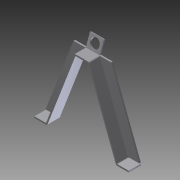
# Autodesk Inventor part: bunny throw base 2
Saved by Autodesk Inventor 2012 (Build 160160000, 160)
## iProperties
Created: 2013-10-11
Part Number: bunny throw base 2
Material: Default
Document SubType Name: Modeling
Designer: Bryce
Density: 1 g/cm^3
Author: Bryce
Autodesk Inventor part; units mm, degrees
ref_plane "YZ Plane" through (0, 0, 0) normal (1, 0, 0) x (0, 1, 0)
ref_plane "XZ Plane" through (0, 0, 0) normal (0, 1, 0) x (-1, 0, 0)
ref_plane "XY Plane" through (0, 0, 0) normal (0, 0, 1) x (1, 0, 0)
sketch "Sketch1" plane through (0, 0, 0) normal (0, 0, 1) x (1, 0, 0)
  line L0 (0, 0) -> (193.675, 0)
  line L1 (84.1375, 152.4) -> (109.5375, 152.4)
  line L2 (84.1375, 152.4) -> (25.9752, 0)
  line L3 (109.5375, 152.4) -> (167.6998, 0)
  line L4 (58.1623, 155.575) -> (0.6059, 4.7625)
  line L5 (135.5127, 155.575) -> (193.0691, 4.7625)
  line L6 (0, 0) -> (0, 3.175)
  line L7 (0, 3.175) -> (23.7885, 3.175)
  line L8 (193.675, 0) -> (193.675, 3.175)
  line L9 (193.675, 3.175) -> (169.8865, 3.175)
  line L10 (169.8865, 3.175) -> (111.7241, 155.575)
  line L11 (111.7241, 155.575) -> (81.9509, 155.575)
  line L12 (81.9509, 155.575) -> (23.7885, 3.175)
  line L13 (58.1623, 155.575) -> (81.9509, 155.575)
  line L14 (111.7241, 155.575) -> (135.5127, 155.575)
  line L15 (0.6059, 4.7625) -> (22.3923, 4.7625)
  line L16 (193.0691, 4.7625) -> (171.2827, 4.7625)
  arc A0 (22.3923, 3.175) -> (22.3923, 4.7625) centre (22.3923, 3.9688) ccw
  arc A1 (171.2827, 4.7625) -> (171.2827, 3.175) centre (171.2827, 3.9688) ccw
  dimension "d0" = 193.675
  dimension "d1" = 25.4
  dimension "d2" = 25.4
  dimension "d3" = 25.4
  dimension "d4" = 3.175
  dimension "d5" = 3.175
  dimension "d6" = 152.4
  dimension "d7" = 1.5875
  dimension "d8" = 1.5875
  dimension "d9" = 1.5875
  constraints: 34 end point, 8 point on line, 4 parallel, 4 perpendicular, 4 point on circle, 4 tangent, 3 collinear, 2 centre point, 2 horizontal alignment, 1 equal length, 1 horizontal, 2 other
  measures "d0" distance of L0.start L0.end
  measures "d1" distance of L1.start L1.end
  measures "d2" distance between parallel lines of L2 L4
  measures "d3" distance between parallel lines of L5 L3
  measures "d4" distance of L0.start L6.end
  measures "d5" distance between parallel lines of L11 L1
  measures "d6" distance between parallel lines of L0 L1
  measures "d7" distance between parallel lines of L7 L15
  measures "d8" distance from line of L10 A1.centre
  measures "d9" distance from line of L12 A0.centre
extrude "Extrusion1" add sketch "Sketch1" along normal blind 25.4 contours L6 L7 L12 L11 L10 L9 L8 L0 L3 L1 L2
extrude "Extrusion2" add sketch "Sketch1" along normal blind 3.175 contours A0 L15 L4 L13 L12 L7 | L9 L10 L14 L5 L16 A1
fillet "Fillet1" radius 1.5875 4 edges at (169.8865, 3.175, 14.2875) (23.7885, 3.175, 14.2875) (84.1375, 152.4, 12.7) (109.5375, 152.4, 12.7)
fillet "Fillet2" radius 3.175 4 edges at (81.9509, 155.575, 14.2875) (111.7241, 155.575, 14.2875) (25.9752, 0, 12.7) (167.6998, 0, 12.7)
ref_plane "Work Plane1" through (96.8375, 0, 0) normal (1, 0, 0) x (0, 0, -1)
sketch "Sketch2" plane through (96.8375, 0, 0) normal (1, 0, 0) x (0, 0, -1)
  line L0 (0, 153.2705) -> (9.1308, 178.3573)
  line L1 (9.1308, 178.3573) -> (6.1473, 179.4432)
  line L2 (6.1473, 179.4432) -> (-2.54, 155.575)
  line L3 (-2.54, 155.575) -> (0, 155.575)
  line L4 (0, 155.575) -> (0, 153.2705)
  line L5 (0, 155.575) -> (0, 4.7625) projected
  line L6 (0, 155.575) -> (-3.175, 155.575) projected
  line L7 (-25.4, 155.575) -> (-3.175, 155.575) projected
  point P0 (0, 0)
  dimension "d16" = 3.175
  dimension "d17" = 110
  dimension "d18" = 25.4
  dimension "d19" = 2.54
  constraints: 10 end point, 3 perpendicular, 2 collinear, 1 horizontal
  measures "d16" distance of L0.end L1.end
  measures "d17" angle of L2 L7
  measures "d18" distance of L1.end L2.end
  measures "d19" distance of L2.end L3.end
extrude "Extrusion3" add sketch "Sketch2" along normal mid plane 28.575
fillet "Fillet3" radius 3.175 1 edges at (96.8375, 153.2705, 0)
sketch "Sketch3" plane through (82.55, 179.4432, -6.1473) normal (0, 0.3420201, 0.9396926) x (1, 0, 0)
  line L0 (28.575, -25.4) -> (28.575, 0) projected
  line L1 (0, 0) -> (28.575, 0) projected
  circle A0 centre (14.2875, -12.7) radius 9.525
  point P0 (-82.55, -170.7239)
  dimension "d23" = 19.05
  dimension "d24" = 14.2875
  dimension "d25" = 12.7
  constraints: 1 centre point
  measures "d23" diameter of A0
  measures "d24" distance from line of L0 A0.centre
  measures "d25" distance from line of L1 A0.centre
extrude "Extrusion4" cut sketch "Sketch3" against normal blind 25.4
equation "\"d5\" = d4"
equation "\"d7\" = 0.5 * d4"
equation "\"d9\" = d8"
body "Solid1"
